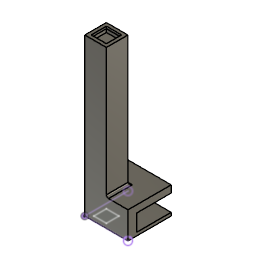
Shoe Rack Bracket v2.2 (Autodesk Fusion 360 design; units mm, degrees)
part number: 2026-02-13-20-43-58-642
Autodesk Fusion 360 part; units mm, degrees
note: some values were not read from the file. Set by a fixed rule: which sketch regions a step uses.
sketch "Sketch1" plane through (0, 0, 0) normal (0, 0, 1) x (1, 0, 0)
  line L0 (0, 0) -> (50.8, 0)
  line L1 (50.8, 0) -> (50.8, 50.8)
  line L2 (50.8, 50.8) -> (0, 50.8)
  line L3 (0, 50.8) -> (0, 0)
  dimension "d1" = 50.8
  dimension "d2" = 50.8
  constraint horizontal L0
  constraint vertical L1
  constraint horizontal L2
  constraint vertical L3
  constraint coincident L0.start L3.end
  measures "d1" distance of L1 L3
  measures "d2" distance of L0 L2
extrude "Extrude1" add sketch "Sketch1" along normal blind 31.75
sketch "Sketch2" plane through (50.8, 0, 0) normal (1, 0, 0) x (0, 1, 0)
  line L0 (0, 0) -> (50.8, 0)
  line L1 (50.8, 0) -> (50.8, 31.75)
  line L2 (50.8, 31.75) -> (0, 31.75)
  line L3 (0, 31.75) -> (0, 0)
  line L4 (50.8, 23.368) -> (10.16, 23.368)
  line L5 (10.16, 23.368) -> (10.16, 3.81)
  line L6 (10.16, 3.81) -> (50.8, 3.81)
  line L7 (50.8, 3.81) -> (50.8, 23.368)
  dimension "d5" = 40.64
  dimension "d6" = 19.558
  dimension "d14" = 3.81
  constraint horizontal L4
  constraint vertical L5
  constraint horizontal L6
  constraint vertical L7
  constraint coincident L1 L4.start
  measures "d5" distance of L5 L7
  measures "d6" distance of L4 L6
  measures "d14" distance of L0 L6
extrude "Extrude2" cut sketch "Sketch2" against normal blind 40.64 contours L1 L4 L5 L6 L7
sketch "Sketch3" plane through (0, 0, 31.75) normal (0, 0, 1) x (-1, 0, 0)
  line L0 (0, -50.8) -> (0, 0)
  line L1 (0, 0) -> (-50.8, 0)
  line L2 (-50.8, 0) -> (-50.8, -50.8)
  line L3 (-50.8, -50.8) -> (0, -50.8)
  line L4 (0, 0) -> (-25.4, 0)
  line L5 (-25.4, 0) -> (-25.4, -25.4)
  line L6 (-25.4, -25.4) -> (0, -25.4)
  line L7 (0, -25.4) -> (0, 0)
  dimension "d10" = 25.4
  dimension "d11" = 25.4
  constraint horizontal L4
  constraint vertical L5
  constraint horizontal L6
  constraint vertical L7
  constraint coincident L0.end L1.start
  measures "d10" distance of L5 L7
  measures "d11" distance of L4 L6
extrude "Extrude3" add sketch "Sketch3" along normal blind 152.4 contours L0 L1 L4 L5 L6 L7
fillet "Fillet1" radius 2.54 2 edges at (25.4, 12.7, 31.75) (12.7, 25.4, 31.75)
sketch "Sketch4" plane through (0, 0, 0) normal (0, 0, -1) x (1, 0, 0)
  line L0 (0, 0) -> (0, -50.8)
  line L1 (0, -50.8) -> (50.8, -50.8)
  line L2 (50.8, -50.8) -> (50.8, 0)
  line L3 (50.8, 0) -> (0, 0)
  line L4 (2.54, -2.54) -> (22.86, -2.54)
  line L5 (22.86, -2.54) -> (22.86, -22.86)
  line L6 (22.86, -22.86) -> (2.54, -22.86)
  line L7 (2.54, -22.86) -> (2.54, -2.54)
  dimension "d17" = 2.54
  dimension "d18" = 2.54
  dimension "d19" = 20.32
  dimension "d20" = 20.32
  constraint horizontal L4
  constraint vertical L5
  constraint horizontal L6
  constraint vertical L7
  measures "d17" distance of L3 L4
  measures "d18" distance of L0 L7
  measures "d19" distance of L5 L7
  measures "d20" distance of L4 L6
sketch "Sketch5" plane through (0, 0, 0) normal (0, 0, -1) x (1, 0, 0)
  line L0 (5.334, -5.334) -> (20.066, -5.334)
  line L1 (20.066, -5.334) -> (20.066, -20.066)
  line L2 (20.066, -20.066) -> (5.334, -20.066)
  line L3 (5.334, -20.066) -> (5.334, -5.334)
  line L4 (0, -50.8) -> (0, 0)
  line L5 (0, 0) -> (50.8, 0)
  dimension "d23" = 14.732
  dimension "d24" = 14.732
  dimension "d39" = 5.334
  dimension "d40" = 5.334
  constraint horizontal L0
  constraint vertical L1
  constraint horizontal L2
  constraint vertical L3
  measures "d23" distance of L0 L2
  measures "d24" distance of L1 L3
  measures "d39" distance of L3 L4
  measures "d40" distance of L0 L5
sketch "Sketch6" plane through (0, 0, 184.15) normal (0, 0, 1) x (-1, 0, 0)
  line L0 (0, -25.4) -> (0, 0)
  line L1 (0, 0) -> (-25.4, 0)
  line L2 (-25.4, 0) -> (-25.4, -25.4)
  line L3 (-25.4, -25.4) -> (0, -25.4)
  line L4 (-5.08, -20.32) -> (-20.32, -20.32)
  line L5 (-20.32, -20.32) -> (-20.32, -5.08)
  line L6 (-20.32, -5.08) -> (-5.08, -5.08)
  line L7 (-5.08, -5.08) -> (-5.08, -20.32)
  dimension "d27" = 5.08
  dimension "d28" = 5.08
  dimension "d29" = 5.08
  dimension "d30" = 15.24
  constraint horizontal L4
  constraint vertical L5
  constraint horizontal L6
  constraint vertical L7
  measures "d27" distance of L0 L7
  measures "d28" distance of L2 L5
  measures "d29" distance of L1 L6
  measures "d30" distance of L4 L6
extrude "Extrude5" cut sketch "Sketch6" against normal blind 5.08 contours L4 L5 L6 L7
fillet "Fillet2" radius 1.27 4 edges at (5.08, 12.7, 184.15) (12.7, 20.32, 184.15) (12.7, 5.08, 184.15) (20.32, 12.7, 184.15)
extrude "Extrude6" add sketch "Sketch5" along normal blind 5.08
equation "d23 = 0.6 in - 0.02 in"
equation "d24 = 0.6 in - 0.02 in"
